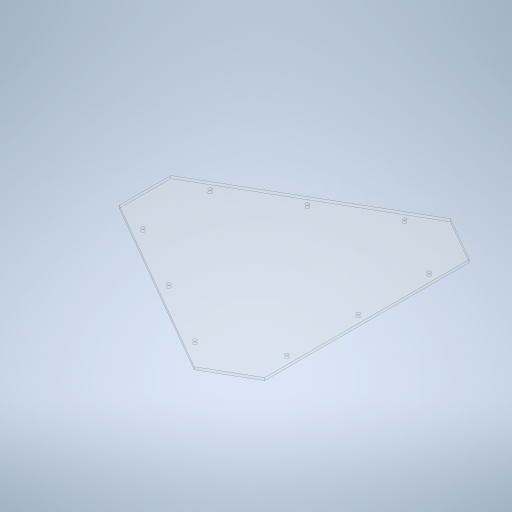
# Autodesk Inventor part: acrylic
Saved by Autodesk Inventor 2024.2 (Build 282272000, 272)
## iProperties
Created: 2024-03-31
Part Number: acrylic
Material: Polycarbonate, Clear
Document SubType Name: Modeling
Designer: Robin
Density: 1.2 g/cm^3
Appearance: Polycarbonate - Clear
Author: Robin
Autodesk Inventor part; units mm, degrees
ref_plane "YZ Plane" through (0, 0, 0) normal (1, 0, 0) x (0, 1, 0)
ref_plane "XZ Plane" through (0, 0, 0) normal (0, 1, 0) x (-1, 0, 0)
ref_plane "XY Plane" through (0, 0, 0) normal (0, 0, 1) x (1, 0, 0)
sketch "Sketch1" plane through (0, 0, 0) normal (0, 1, 0) x (-1, 0, 0)
  line L0 (299.6448, 0) -> (0, 173)
  line L1 (0, 173) -> (0, -173)
  line L2 (0, -173) -> (299.6448, 0)
  line L3 (249.4153, 29) -> (249.4153, -29)
  line L4 (50.2295, -144) -> (0, -115)
  line L5 (50.2295, 144) -> (0, 115)
  point P0 (0, 0)
  point P1 (0, 0)
  dimension "d0" = 60
  dimension "d1" = 60
  dimension "d3" = 58
  dimension "d5" = 60
  dimension "d6" = 60
  dimension "d7" = 58
  dimension "d8" = 58
  dimension "d34" = 230
  constraints: 12 end point, 6 point on line, 2 vertical, 1 horizontal alignment, 1 midpoint, 1 vertical alignment
  measures "d0" angle of L0 L1
  measures "d1" angle of L1 L2
  measures "d3" distance of L3.start L3.end
  measures "d5" angle of L3 L5
  measures "d6" angle of L4 L5
  measures "d7" distance of L5.start L5.end
  measures "d8" distance of L4.start L4.end
  measures "d34" distance of L3.end L4.start
extrude "Extrusion1" add sketch "Sketch1" along normal blind 3 contours L3 L2 L4 L1 L5 L0
sketch "Sketch2" plane through (0, 3, 0) normal (0, 1, 0) x (1, 0, 0)
  line L0 (0, -115) -> (0, 115) projected
  point P0 (0, 0)
  point P1 (-10, -80)
  point P2 (-10, 0)
  point P3 (-10, 80)
  point P4 (0, 0)
  point P5 (0, 0)
  point P6 (0, 0)
  dimension "d11" = 10
  dimension "d12" = 80
  dimension "d13" = 80
  dimension "d14" = 10
  dimension "d15" = 10
  constraints: 3 midpoint, 1 horizontal alignment
  measures "d11" distance of point (0, 0) point (-10, 0)
  measures "d12" distance of point (-10, 0) point (-10, -80)
  measures "d13" vertical distance of point (0, 0) point (-10, 80)
  measures "d14" distance from line of L0 point (-10, -80)
  measures "d15" distance from line of L0 point (-10, 80)
hole "Hole1" at (-10, 3, 80) at (-10, 3, 0) at (-10, 3, -80) direction (0, -1, 0) diameter 4 end through all
sketch "Sketch3" plane through (0, 3, 0) normal (0, 1, 0) x (1, 0, 0)
  line L0 (-214.1044, -37.8397) -> (-75.5404, -117.8397)
  line L1 (-75.5404, 117.8397) -> (-214.1044, 37.8397)
  line L2 (-50.2295, 144) -> (-249.4153, 29) projected
  line L3 (-249.4153, -29) -> (-50.2295, -144) projected
  line L4 (-144.8224, -77.8397) -> (-149.8224, -86.5)
  line L5 (-144.8224, 77.8397) -> (-149.8224, 86.5)
  line L6 (-50.2295, 144) -> (-249.4153, 29) projected
  point P0 (0, 0)
  dimension "d23" = 160
  dimension "d24" = 160
  dimension "d25" = 10
  dimension "d26" = 10
  constraints: 8 end point, 6 coincident, 4 midpoint, 2 parallel, 2 perpendicular
  measures "d23" distance of L1.start L1.end
  measures "d24" distance of L0.start L0.end
  measures "d25" distance between parallel lines of L3 L0
  measures "d26" distance between parallel lines of L2 L1
hole "Hole2" at (-214.1044, 3, -37.8397) at (-144.8224, 3, -77.8397) at (-75.5404, 3, -117.8397) at (-214.1044, 3, 37.8397) at (-144.8224, 3, 77.8397) at (-75.5404, 3, 117.8397) direction (0, -1, 0) diameter 4 end through all
body "Solid1"
